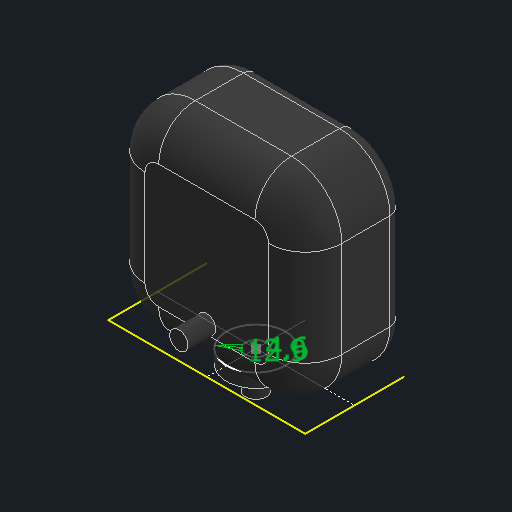
# Autodesk Inventor part: camera
Saved by Autodesk Inventor 2026.1 (Build 301233020, 233B)
## iProperties
Created: 2025-12-04
Part Number: camera
Material: 고무, 검은색
Document SubType Name: Modeling
Designer: jaewook
Density: 0.93 g/cm^3
Appearance: 고무 - 검은색
Author: jaewook
Autodesk Inventor part; units mm, degrees
ref_plane "YZ Plane" through (0, 0, 0) normal (1, 0, 0) x (0, 1, 0)
ref_plane "XZ Plane" through (0, 0, 0) normal (0, 1, 0) x (-1, 0, 0)
ref_plane "XY Plane" through (0, 0, 0) normal (0, 0, 1) x (1, 0, 0)
sketch "스케치1" plane through (0, 0, 0) normal (0, 0, 1) x (1, 0, 0)
  line L0 (21.5, -21.5) -> (-21.5, -21.5)
  line L1 (-21.5, -21.5) -> (-21.5, 21.5)
  line L2 (-21.5, 21.5) -> (21.5, 21.5)
  line L3 (21.5, 21.5) -> (21.5, -21.5)
  line L4 (21.5, -21.5) -> (-21.5, 21.5) construction
  line L5 (-21.5, -21.5) -> (21.5, 21.5) construction
  point P0 (0, 0)
  dimension "d0" = 43
  dimension "d1" = 43
  constraints: 12 end point, 2 midpoint, 2 parallel, 1 horizontal, 1 perpendicular
  measures "d0" distance of L1.end L2.end
  measures "d1" distance of L0.end L1.end
extrude "돌출1" add sketch "스케치1" along normal blind 21.5
sketch "스케치2" plane through (0, 0, 0) normal (0, 0, -1) x (-1, 0, 0)
  circle A0 centre (0, 0) radius 11.2
  dimension "d4" = 22.4
  constraints: 1 centre point, 1 coincident
  measures "d4" diameter of A0
extrude "돌출2" add sketch "스케치2" along normal blind 6.1
sketch "스케치3" plane through (0, 0, 21.5) normal (0, 0, 1) x (1, 0, 0)
  line L0 (-21.5, -21.5) -> (21.5, -21.5) projected
  circle A0 centre (0, -11.5) radius 2
  point P0 (0, 0)
  dimension "d7" = 4
  dimension "d8" = 10
  constraints: 1 centre point, 1 vertical alignment
  measures "d7" diameter of A0
  measures "d8" distance from line of L0 A0.centre
extrude "돌출3" add sketch "스케치3" along normal blind 6.1
sketch "스케치4" plane through (-21.5, -21.5, 0) normal (0, -1, 0) x (1, 0, 0)
  line L0 (43, 0) -> (43, 21.5) projected
  line L1 (0, 21.5) -> (43, 21.5) projected
  line L2 (0, 0) -> (0, 21.5) projected
  line L3 (43, 10.75) -> (0, 10.75) construction
  line L4 (21.5, 0) -> (21.5, 21.5) construction
  circle A0 centre (21.5, 10.75) radius 6.45
  circle A1 centre (21.5, 10.75) radius 2.3
  dimension "d11" = 12.9
  dimension "d12" = 4.6
  constraints: 4 end point, 4 midpoint, 2 centre point, 1 coincident
  measures "d11" diameter of A0
  measures "d12" diameter of A1
extrude "돌출4" add sketch "스케치4" along normal blind 8 contours A1
extrude "돌출5" add sketch "스케치4" along normal blind 3
fillet "모깎기1" radius 11 4 edges at (-21.5, -21.5, 10.75) (21.5, -21.5, 10.75) (-21.5, 21.5, 10.75) (21.5, 21.5, 10.75)
fillet "모깎기2" radius 8 8 edges at (0, -21.5, 21.5) (-18.2782, -18.2782, 21.5) (-21.5, 0, 21.5) (-18.2782, 18.2782, 21.5) (0, 21.5, 21.5) (18.2782, 18.2782, 21.5) (21.5, 0, 21.5) (18.2782, -18.2782, 21.5)
fillet "모깎기3" radius 3 8 edges at (21.5, 0, 0) (18.2782, 18.2782, 0) (0, 21.5, 0) (-18.2782, 18.2782, 0) (-21.5, 0, 0) (-18.2782, -18.2782, 0) (0, -21.5, 0) (18.2782, -18.2782, 0)
equation "\"d1\" = d0"
